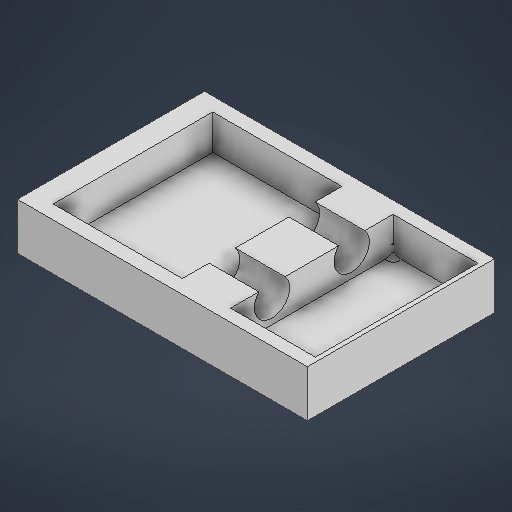
# Autodesk Inventor part: Bottom
Saved by Autodesk Inventor 2026.2 (Build 302298010, 298A)
## iProperties
Created: 2026-09-18
Part Number: Bottom
Material: Ogólny
Document SubType Name: Modeling
Designer: Rozkurwiator
Density: 1 g/cm^3
Appearance: Domyślna
Author: Rozkurwiator
Autodesk Inventor part; units mm, degrees
ref_plane "YZ Plane" through (0, 0, 0) normal (1, 0, 0) x (0, 1, 0)
ref_plane "XZ Plane" through (0, 0, 0) normal (0, 1, 0) x (-1, 0, 0)
ref_plane "XY Plane" through (0, 0, 0) normal (0, 0, 1) x (1, 0, 0)
sketch "Szkic1" plane through (0, 0, 0) normal (0, 1, 0) x (-1, 0, 0)
  line L0 (-60.1, 40) -> (60.1, 40)
  line L1 (60.1, 40) -> (60.1, -40)
  line L2 (60.1, -40) -> (-60.1, -40)
  line L3 (-60.1, -40) -> (-60.1, 40)
  line L4 (-60.1, 40) -> (60.1, -40) construction
  line L5 (60.1, 40) -> (-60.1, -40) construction
  line L6 (0, 0) -> (-42, 0)
  line L7 (0, 0) -> (42, 0) construction
  line L8 (-60.1355, -34.75) -> (-23.8645, -34.75)
  line L9 (-23.8645, -34.75) -> (-23.8645, 34.75)
  line L10 (-23.8645, 34.75) -> (-60.1355, 34.75)
  line L11 (-60.1355, 34.75) -> (-60.1355, -34.75)
  line L12 (-60.1355, -34.75) -> (-23.8645, 34.75) construction
  line L13 (-23.8645, -34.75) -> (-60.1355, 34.75) construction
  line L14 (0, 0) -> (25, 0)
  line L15 (52.6, 34.1) -> (-2.6, 34.1)
  line L16 (-2.6, 34.1) -> (-2.6, -34.1)
  line L17 (-2.6, -34.1) -> (52.6, -34.1)
  line L18 (52.6, -34.1) -> (52.6, 34.1)
  line L19 (52.6, 34.1) -> (-2.6, -34.1) construction
  line L20 (-2.6, 34.1) -> (52.6, -34.1) construction
  line L21 (-62, -40) -> (62, -40)
  line L22 (62, -40) -> (62, 40)
  line L23 (62, 40) -> (-62, 40)
  line L24 (-62, 40) -> (-62, -40)
  line L25 (-62, -40) -> (62, 40) construction
  line L26 (62, -40) -> (-62, 40) construction
  dimension "d0" = 120.2
  dimension "d1" = 80
  dimension "d2" = 42
  dimension "d3" = 180
  dimension "d4" = 36.271
  dimension "d5" = 69.5
  dimension "d6" = 25
  dimension "d7" = 55.2
  dimension "d8" = 68.2
  dimension "d9" = 124
  dimension "d10" = 80
  constraints: 54 end point, 8 midpoint, 8 parallel, 6 horizontal, 4 perpendicular, 1 collinear, 1 point on line
  measures "d0" distance of L0.start L0.end
  measures "d1" distance of L0.end L1.end
  measures "d2" distance of L6.start L6.end
  measures "d3" angle of L6 L7
  measures "d4" distance of L10.end L9.end
  measures "d5" distance of L9.end L8.end
  measures "d6" distance of L6.start L14.end
  measures "d7" distance of L17.end L16.end
  measures "d8" distance of L16.end L15.end
  measures "d9" distance of L23.end L22.end
  measures "d10" distance of L22.end L21.end
extrude "Wyciągnięcie proste1" add sketch "Szkic1" against normal blind 5 contours L0 L1 L2 L3 L8 L9 L10 | L3 L10 L11 L8 L21 L24 L23 | L23 L22 L21 L1 | L10 L9 L8 L3 | L3 L8 L11 L10 | L18 L17 L16 L15
extrude "Wyciągnięcie proste2" add sketch "Szkic1" along normal blind 15 contours L0 L1 L2 L3 L8 L9 L10 | L3 L10 L11 L8 L21 L24 L23 | L23 L22 L21 L1
sketch "Szkic2" plane through (23.8645, 0, -34.75) normal (1, 0, 0) x (0, 0, -1)
  line L0 (-68.85, 0) -> (-68.85, 15) projected
  line L1 (-68.85, 15) -> (-0.65, 15) projected
  line L2 (-68.85, 15) -> (-0.65, 15)
  line L3 (-68.85, 15) -> (-34.75, 15)
  line L4 (-34.75, 15) -> (-34.75, 0)
  line L5 (-51.8, 15) -> (-51.8, 10)
  line L6 (-51.8, 15) -> (-46.8, 15) construction
  circle A0 centre (-51.8, 10) radius 7.5
  circle A1 centre (-17.7, 10) radius 7.5
  point P0 (-23.2902, 15)
  point P1 (-12.1098, 15)
  point P2 (-57.3902, 15)
  point P3 (-46.2098, 15)
  dimension "d15" = 5
  dimension "d16" = 90
  dimension "d17" = 15
  constraints: 10 end point, 2 centre point, 2 midpoint, 2 vertical, 1 coincident, 1 collinear, 1 horizontal, 1 perpendicular, 1 symmetric about line, 1 other
  measures "d15" distance of L5.start L5.end
  measures "d16" angle of L5 L6
  measures "d17" diameter of A0
extrude "Wyciągnięcie proste3" cut sketch "Szkic2" against normal blind 25 contours L1 A0 | L1 A1 picked at (-51.8096, 6.7032) picked at (-18.0065, 10.8522)
sketch "Szkic3" plane through (0, 0, 0) normal (0, 1, 0) x (1, 0, 0)
  line L0 (23.8645, 34.75) -> (60.1355, 34.75) construction
  line L1 (60.1355, 34.75) -> (60.1355, -34.75) construction
  line L2 (60.1355, -34.75) -> (23.8645, 34.75) construction
  line L3 (60.1355, -34.75) -> (23.8645, -34.75) construction
  line L4 (60.1355, 34.75) -> (23.8645, -34.75) construction
  line L5 (60.1355, 34.75) -> (23.8645, 34.75) construction
  line L6 (23.8645, 34.75) -> (23.8645, -34.75) construction
  line L7 (23.8645, -34.75) -> (60.1355, -34.75) construction
  line L8 (60.1355, -34.75) -> (60.1355, 34.75) construction
  line L9 (60.1355, 34.75) -> (23.8645, -34.75) construction
  line L10 (23.8645, 34.75) -> (60.1355, -34.75) construction
  line L11 (23.8645, -34.75) -> (24.9252, -33.6893) construction
  line L12 (23.8645, -34.75) -> (25.3645, -34.75) construction
  circle A0 centre (24.9252, -33.6893) radius 0.4
  line L13 (23.8645, 0) -> (60.1355, 0) construction
  line L14 (42, -34.75) -> (42, 34.75) construction
  circle A1 centre (24.9252, 33.6893) radius 0.4
  circle A2 centre (59.0748, 33.6893) radius 0.4
  circle A3 centre (59.0748, -33.6893) radius 0.4
  point P0 (0, 0)
  point P1 (42, 0)
  dimension "d20" = 1.5
  dimension "d21" = 45
  dimension "d22" = 0.8
  constraints: 24 end point, 7 midpoint, 4 centre point, 3 symmetric about line, 2 horizontal, 2 parallel, 1 coincident, 1 equal length, 1 perpendicular, 3 other
  measures "d20" distance of L3.end L11.end
  measures "d21" angle of L12 L11
  measures "d22" diameter of A0
extrude "Wyciągnięcie proste4" add sketch "Szkic3" along normal blind 5
fillet "Zaokrąglenie1" radius 2 4 edges at (24.5252, 0, 33.6893) (58.6748, 0, 33.6893) (24.5252, 0, -33.6893) (58.6748, 0, -33.6893)
